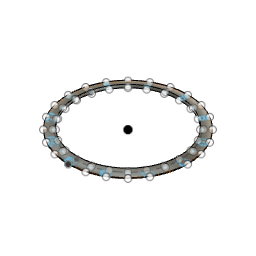
Bezel_Insert v4 (Autodesk Fusion 360 design; units mm, degrees)
Autodesk Fusion 360 part; units mm, degrees
note: some values were not read from the file. Set by a fixed rule: which sketch regions a step uses.
sketch "Sketch1" plane through (0, 0, 0) normal (0, 1, 0) x (1, 0, 0)
  line L0 (0, 0) -> (18.0594, 0) construction
  line L1 (18.0594, 0) -> (15.4305, 0)
  line L2 (18.0594, 0) -> (18.0594, -0.2032)
  arc A0 (15.5217, -0.9118) -> (18.0594, -0.2032) centre (15.4613, 4.2031) ccw
  line L3 (15.4305, 0) -> (15.5217, 0)
  line L4 (15.5217, 0) -> (15.5217, -0.9118)
  dimension "d2" = 15.4305
  dimension "d3" = 0.2032
  dimension "d5" = 2.6289
  constraint coincident L0.start origin
  constraint horizontal L0
  constraint vertical L2
  constraint coincident L1 L3.end
  constraint coincident L0 L3.end
  constraint perpendicular L3 L4
  measures "d2" distance of L0.start L1.end
  measures "d3" distance of L0.end L2.end
  measures "d5" distance of L0.end L1.end
revolve "Revolve1" add sketch "Sketch1" angle 360 about axis through (0, 0, 1.75) along (0, 0, 1)
sketch "Sketch2" plane through (0, 0, 0) normal (0, 0, -1) x (1, 0, 0)
  circle A0 centre (0, 0) radius 15.5217 construction
  circle A1 centre (0, 0) radius 18.0594 construction
  line L0 (0, 18.0594) -> (0, 15.5217) construction
  line L1 (-4.6741, 17.444) -> (-4.0173, 14.9928) construction
  line L2 (-9.0297, 15.6399) -> (-7.7609, 13.4422) construction
  line L3 (-12.7699, 12.7699) -> (-10.9755, 10.9755) construction
  line L4 (-15.6399, 9.0297) -> (-13.4422, 7.7609) construction
  line L5 (-17.444, 4.6741) -> (-14.9928, 4.0173) construction
  line L6 (-18.0594, 0) -> (-15.5217, 0) construction
  line L7 (-17.444, -4.6741) -> (-14.9928, -4.0173) construction
  line L8 (-15.6399, -9.0297) -> (-13.4422, -7.7609) construction
  line L9 (-12.7699, -12.7699) -> (-10.9755, -10.9755) construction
  line L10 (-9.0297, -15.6399) -> (-7.7609, -13.4422) construction
  line L11 (-4.6741, -17.444) -> (-4.0173, -14.9928) construction
  line L12 (0, -18.0594) -> (0, -15.5217) construction
  line L13 (4.6741, -17.444) -> (4.0173, -14.9928) construction
  line L14 (9.0297, -15.6399) -> (7.7609, -13.4422) construction
  line L15 (12.7699, -12.7699) -> (10.9755, -10.9755) construction
  line L16 (15.6399, -9.0297) -> (13.4422, -7.7609) construction
  line L17 (17.444, -4.6741) -> (14.9928, -4.0173) construction
  line L18 (18.0594, 0) -> (15.5217, 0) construction
  line L19 (17.444, 4.6741) -> (14.9928, 4.0173) construction
  line L20 (15.6399, 9.0297) -> (13.4422, 7.7609) construction
  line L21 (12.7699, 12.7699) -> (10.9755, 10.9755) construction
  line L22 (9.0297, 15.6399) -> (7.7609, 13.4422) construction
  line L23 (4.6741, 17.444) -> (4.0173, 14.9928) construction
  line L24 (-15.2263, 8.2238) -> (-15.3043, 8.2626)
  line L25 (-15.3043, 8.2626) -> (-15.499, 8.2622)
  line L26 (-15.499, 8.2622) -> (-15.6158, 8.2231)
  line L27 (-15.6158, 8.2231) -> (-15.7714, 8.1059)
  line L28 (-15.7714, 8.1059) -> (-15.9265, 7.794)
  line L29 (-15.9265, 7.794) -> (-15.9261, 7.5993)
  line L30 (-15.9261, 7.5993) -> (-15.887, 7.4825)
  line L31 (-15.887, 7.4825) -> (-15.7698, 7.327)
  line L32 (-15.7698, 7.327) -> (-15.6139, 7.2494)
  line L33 (-15.6139, 7.2494) -> (-15.4191, 7.2498)
  line L34 (-15.4191, 7.2498) -> (-15.1077, 7.2894)
  line L35 (-15.1077, 7.2894) -> (-13.94, 7.6811)
  line L36 (-13.94, 7.6811) -> (-14.4831, 6.5896)
  line L37 (-14.1837, 9.8328) -> (-14.2562, 9.8809)
  line L38 (-14.2562, 9.8809) -> (-14.4495, 9.9048)
  line L39 (-14.4495, 9.9048) -> (-14.5702, 9.8804)
  line L40 (-14.5702, 9.8804) -> (-14.7391, 9.7835)
  line L41 (-14.7391, 9.7835) -> (-14.9319, 9.4934)
  line L42 (-14.9319, 9.4934) -> (-14.9557, 9.3001)
  line L43 (-14.9557, 9.3001) -> (-14.9314, 9.1794)
  line L44 (-14.9314, 9.1794) -> (-14.8345, 9.0105)
  line L45 (-14.8345, 9.0105) -> (-14.6894, 8.9141)
  line L46 (-14.6894, 8.9141) -> (-14.4962, 8.8903)
  line L47 (-14.4962, 8.8903) -> (-14.1822, 8.8908)
  line L48 (-14.1822, 8.8908) -> (-12.9749, 9.1343)
  line L49 (-9.6456, 14.8241) -> (-9.3826, 14.9058)
  line L50 (-9.3826, 14.9058) -> (-9.0888, 14.7952)
  line L51 (-9.0888, 14.7952) -> (-8.764, 14.4924)
  line L52 (-8.764, 14.4924) -> (-8.6116, 14.2802)
  line L53 (-8.6116, 14.2802) -> (-8.4282, 13.8757)
  line L54 (-8.4282, 13.8757) -> (-8.4173, 13.5619)
  line L55 (-8.4173, 13.5619) -> (-8.5787, 13.3388)
  line L56 (-8.5787, 13.3388) -> (-8.7201, 13.2372)
  line L57 (-8.7201, 13.2372) -> (-8.9831, 13.1555)
  line L58 (-8.9831, 13.1555) -> (-9.277, 13.266)
  line L59 (-9.277, 13.266) -> (-9.6018, 13.5689)
  line L60 (-9.6018, 13.5689) -> (-9.7542, 13.7811)
  line L61 (-9.7542, 13.7811) -> (-9.9375, 14.1855)
  line L62 (-9.9375, 14.1855) -> (-9.9485, 14.4993)
  line L63 (-9.9485, 14.4993) -> (-9.7871, 14.7225)
  line L64 (-9.7871, 14.7225) -> (-9.6456, 14.8241)
  line L65 (-7.3643, 15.6598) -> (-7.406, 15.7363)
  line L66 (-7.406, 15.7363) -> (-7.5657, 15.8477)
  line L67 (-7.5657, 15.8477) -> (-7.6838, 15.8825)
  line L68 (-7.6838, 15.8825) -> (-7.8784, 15.8758)
  line L69 (-7.8784, 15.8758) -> (-8.1844, 15.7093)
  line L70 (-8.1844, 15.7093) -> (-8.2958, 15.5496)
  line L71 (-8.2958, 15.5496) -> (-8.3307, 15.4315)
  line L72 (-8.3307, 15.4315) -> (-8.3239, 15.2369)
  line L73 (-8.3239, 15.2369) -> (-8.2407, 15.0839)
  line L74 (-8.2407, 15.0839) -> (-8.081, 14.9725)
  line L75 (-8.081, 14.9725) -> (-7.8031, 14.8262)
  line L76 (-7.8031, 14.8262) -> (-6.622, 14.4774)
  line L77 (-6.622, 14.4774) -> (-7.693, 13.8948)
  line L78 (-0.8834, 17.6919) -> (-0.6167, 17.6234)
  line L79 (-0.6167, 17.6234) -> (-0.5176, 17.4558)
  line L80 (-0.5176, 17.4558) -> (-0.5053, 17.2821)
  line L81 (-0.5053, 17.2821) -> (-0.5799, 17.1022)
  line L82 (-0.5799, 17.1022) -> (-0.7475, 17.0031)
  line L83 (-0.7475, 17.0031) -> (-1.0889, 16.8917)
  line L84 (-1.0889, 16.8917) -> (-1.3434, 16.7864)
  line L85 (-1.3434, 16.7864) -> (-1.5049, 16.6004)
  line L86 (-1.5049, 16.6004) -> (-1.5795, 16.4206)
  line L87 (-1.5795, 16.4206) -> (-1.5611, 16.16)
  line L88 (-1.5611, 16.16) -> (-1.462, 15.9924)
  line L89 (-1.462, 15.9924) -> (-1.369, 15.9116)
  line L90 (-1.369, 15.9116) -> (-1.1022, 15.8431)
  line L91 (-1.1022, 15.8431) -> (-0.7547, 15.8677)
  line L92 (-0.7547, 15.8677) -> (-0.5003, 15.9729)
  line L93 (-0.5003, 15.9729) -> (-0.4195, 16.0659)
  line L94 (-0.4195, 16.0659) -> (-0.3449, 16.2458)
  line L95 (-0.3449, 16.2458) -> (-0.3633, 16.5064)
  line L96 (-0.3633, 16.5064) -> (-0.4624, 16.674)
  line L97 (-0.4624, 16.674) -> (-0.6484, 16.8355)
  line L98 (-0.6484, 16.8355) -> (-0.9152, 16.904)
  line L99 (-0.9152, 16.904) -> (-1.2688, 16.9663)
  line L100 (-1.2688, 16.9663) -> (-1.4486, 17.0409)
  line L101 (-1.4486, 17.0409) -> (-1.5478, 17.2085)
  line L102 (-1.5478, 17.2085) -> (-1.56, 17.3823)
  line L103 (-1.56, 17.3823) -> (-1.4854, 17.5621)
  line L104 (-1.4854, 17.5621) -> (-1.2309, 17.6674)
  line L105 (-1.2309, 17.6674) -> (-0.8834, 17.6919)
  line L106 (0.9655, 17.4038) -> (0.7154, 17.6757)
  line L107 (0.7154, 17.6757) -> (0.639, 15.8485)
  line L108 (7.357, 15.7798) -> (7.5057, 15.9056)
  line L109 (7.5057, 15.9056) -> (7.7801, 15.8828)
  line L110 (7.7801, 15.8828) -> (7.9402, 15.8142)
  line L111 (7.9402, 15.8142) -> (8.1461, 15.6313)
  line L112 (8.1461, 15.6313) -> (8.2033, 15.3225)
  line L113 (8.2033, 15.3225) -> (8.1118, 14.888)
  line L114 (8.1118, 14.888) -> (7.9404, 14.4877)
  line L115 (7.9404, 14.4877) -> (7.7231, 14.2018)
  line L116 (7.7231, 14.2018) -> (7.4944, 14.1103)
  line L117 (7.4944, 14.1103) -> (7.22, 14.1332)
  line L118 (7.22, 14.1332) -> (7.1399, 14.1675)
  line L119 (7.1399, 14.1675) -> (6.9341, 14.3504)
  line L120 (6.9341, 14.3504) -> (6.8426, 14.5791)
  line L121 (6.8426, 14.5791) -> (6.8654, 14.8535)
  line L122 (6.8654, 14.8535) -> (6.8997, 14.9336)
  line L123 (6.8997, 14.9336) -> (7.0827, 15.1394)
  line L124 (7.0827, 15.1394) -> (7.3113, 15.2309)
  line L125 (7.3113, 15.2309) -> (7.5858, 15.2081)
  line L126 (7.5858, 15.2081) -> (7.6658, 15.1738)
  line L127 (7.6658, 15.1738) -> (7.8717, 14.9909)
  line L128 (7.8717, 14.9909) -> (7.9632, 14.7622)
  line L129 (7.9632, 14.7622) -> (7.9404, 14.4877)
  line L130 (9.5325, 14.6777) -> (9.4346, 15.034)
  line L131 (9.4346, 15.034) -> (8.5306, 13.4442)
  line L132 (14.7542, 9.7576) -> (14.2009, 8.3652)
  line L133 (14.2009, 8.3652) -> (13.4935, 9.4633)
  line L134 (14.7542, 9.7576) -> (13.2168, 8.7672)
  line L135 (15.6269, 7.632) -> (15.745, 7.9821)
  line L136 (15.745, 7.9821) -> (14.1064, 7.1701)
  line L137 (17.3368, 0.2982) -> (17.4239, 0.3002)
  line L138 (17.4239, 0.3002) -> (17.5959, 0.3914)
  line L139 (17.5959, 0.3914) -> (17.6809, 0.4805)
  line L140 (17.6809, 0.4805) -> (17.7639, 0.6567)
  line L141 (17.7639, 0.6567) -> (17.7557, 1.005)
  line L142 (17.7557, 1.005) -> (17.6645, 1.177)
  line L143 (17.6645, 1.177) -> (17.5754, 1.262)
  line L144 (17.5754, 1.262) -> (17.3992, 1.345)
  line L145 (17.3992, 1.345) -> (17.2251, 1.3409)
  line L146 (17.2251, 1.3409) -> (17.053, 1.2497)
  line L147 (17.053, 1.2497) -> (16.7959, 1.0694)
  line L148 (16.7959, 1.0694) -> (15.9459, 0.1782)
  line L149 (15.9459, 0.1782) -> (15.9171, 1.3971)
  line L150 (17.3895, -1.1768) -> (17.6728, -0.9396)
  line L151 (17.6728, -0.9396) -> (15.8512, -0.7778)
  line L152 (15.7537, -8.1665) -> (15.5641, -8.3662)
  line L153 (15.5641, -8.3662) -> (15.2536, -8.4132)
  line L154 (15.2536, -8.4132) -> (14.8223, -8.3074)
  line L155 (14.8223, -8.3074) -> (14.5857, -8.1967)
  line L156 (14.5857, -8.1967) -> (14.2283, -7.9332)
  line L157 (14.2283, -7.9332) -> (14.0655, -7.6647)
  line L158 (14.0655, -7.6647) -> (14.0974, -7.3911)
  line L159 (14.0974, -7.3911) -> (14.1713, -7.2334)
  line L160 (14.1713, -7.2334) -> (14.3609, -7.0337)
  line L161 (14.3609, -7.0337) -> (14.6714, -6.9867)
  line L162 (14.6714, -6.9867) -> (15.1027, -7.0925)
  line L163 (15.1027, -7.0925) -> (15.3393, -7.2032)
  line L164 (15.3393, -7.2032) -> (15.6967, -7.4667)
  line L165 (15.6967, -7.4667) -> (15.8595, -7.7352)
  line L166 (15.8595, -7.7352) -> (15.8276, -8.0088)
  line L167 (15.8276, -8.0088) -> (15.7537, -8.1665)
  line L168 (14.5652, -9.7204) -> (14.9245, -9.6342)
  line L169 (14.9245, -9.6342) -> (13.3655, -8.6782)
  line L170 (8.7046, -15.4101) -> (8.4366, -15.4732)
  line L171 (8.4366, -15.4732) -> (8.271, -15.3707)
  line L172 (8.271, -15.3707) -> (8.1795, -15.2225)
  line L173 (8.1795, -15.2225) -> (8.1621, -15.0286)
  line L174 (8.1621, -15.0286) -> (8.2646, -14.863)
  line L175 (8.2646, -14.863) -> (8.5153, -14.6059)
  line L176 (8.5153, -14.6059) -> (8.6918, -14.3946)
  line L177 (8.6918, -14.3946) -> (8.7486, -14.1549)
  line L178 (8.7486, -14.1549) -> (8.7312, -13.9609)
  line L179 (8.7312, -13.9609) -> (8.594, -13.7386)
  line L180 (8.594, -13.7386) -> (8.4284, -13.6361)
  line L181 (8.4284, -13.6361) -> (8.3085, -13.6078)
  line L182 (8.3085, -13.6078) -> (8.0405, -13.6709)
  line L183 (8.0405, -13.6709) -> (7.744, -13.8539)
  line L184 (7.744, -13.8539) -> (7.5675, -14.0652)
  line L185 (7.5675, -14.0652) -> (7.5391, -14.185)
  line L186 (7.5391, -14.185) -> (7.5565, -14.379)
  line L187 (7.5565, -14.379) -> (7.6937, -14.6013)
  line L188 (7.6937, -14.6013) -> (7.8593, -14.7038)
  line L189 (7.8593, -14.7038) -> (8.099, -14.7605)
  line L190 (8.099, -14.7605) -> (8.3671, -14.6974)
  line L191 (8.3671, -14.6974) -> (8.7092, -14.5885)
  line L192 (8.7092, -14.5885) -> (8.9032, -14.5711)
  line L193 (8.9032, -14.5711) -> (9.0688, -14.6736)
  line L194 (9.0688, -14.6736) -> (9.1603, -14.8218)
  line L195 (9.1603, -14.8218) -> (9.1776, -15.0158)
  line L196 (9.1776, -15.0158) -> (9.0011, -15.2271)
  line L197 (9.0011, -15.2271) -> (8.7046, -15.4101)
  line L198 (0.5376, -17.3918) -> (0.4634, -17.5718)
  line L199 (0.4634, -17.5718) -> (0.2092, -17.6777)
  line L200 (0.2092, -17.6777) -> (0.0355, -17.6904)
  line L201 (0.0355, -17.6904) -> (-0.2314, -17.6225)
  line L202 (-0.2314, -17.6225) -> (-0.4241, -17.3746)
  line L203 (-0.4241, -17.3746) -> (-0.5427, -16.9467)
  line L204 (-0.5427, -16.9467) -> (-0.5744, -16.5124)
  line L205 (-0.5744, -16.5124) -> (-0.5129, -16.1587)
  line L206 (-0.5129, -16.1587) -> (-0.3518, -15.9723)
  line L207 (-0.3518, -15.9723) -> (-0.0976, -15.8664)
  line L208 (-0.0976, -15.8664) -> (-0.0108, -15.8601)
  line L209 (-0.0108, -15.8601) -> (0.2561, -15.9279)
  line L210 (0.2561, -15.9279) -> (0.4425, -16.0889)
  line L211 (0.4425, -16.0889) -> (0.5484, -16.3432)
  line L212 (0.5484, -16.3432) -> (0.5547, -16.43)
  line L213 (0.5547, -16.43) -> (0.4869, -16.6969)
  line L214 (0.4869, -16.6969) -> (0.3259, -16.8833)
  line L215 (0.3259, -16.8833) -> (0.0717, -16.9892)
  line L216 (0.0717, -16.9892) -> (-0.0152, -16.9955)
  line L217 (-0.0152, -16.9955) -> (-0.2821, -16.9277)
  line L218 (-0.2821, -16.9277) -> (-0.4685, -16.7667)
  line L219 (-0.4685, -16.7667) -> (-0.5744, -16.5124)
  line L220 (-8.7289, -15.4091) -> (-8.9167, -13.9226)
  line L221 (-8.9167, -13.9226) -> (-7.767, -14.5426)
  line L222 (-8.7289, -15.4091) -> (-7.8609, -13.7994)
  line L223 (-15.2459, -8.1332) -> (-15.322, -8.1756)
  line L224 (-15.322, -8.1756) -> (-15.4316, -8.3365)
  line L225 (-15.4316, -8.3365) -> (-15.4653, -8.455)
  line L226 (-15.4653, -8.455) -> (-15.4565, -8.6495)
  line L227 (-15.4565, -8.6495) -> (-15.2868, -8.9538)
  line L228 (-15.2868, -8.9538) -> (-15.1259, -9.0634)
  line L229 (-15.1259, -9.0634) -> (-15.0074, -9.0971)
  line L230 (-15.0074, -9.0971) -> (-14.8129, -9.0883)
  line L231 (-14.8129, -9.0883) -> (-14.6608, -9.0034)
  line L232 (-14.6608, -9.0034) -> (-14.5511, -8.8425)
  line L233 (-14.5511, -8.8425) -> (-14.4078, -8.5631)
  line L234 (-14.4078, -8.5631) -> (-14.0715, -7.3784)
  line L235 (-14.0715, -7.3784) -> (-13.4775, -8.4431)
  line L236 (-12.9749, 9.1343) -> (-13.6246, 8.0624)
  circle A2 centre (0, 0) radius 15.748 construction
  line L237 (17.444, 4.6741) -> (17.2214, 4.6145) construction
  circle A3 centre (0, 0) radius 17.8289 construction
  line L238 (-17.682, -0.7501) -> (-15.9065, 0)
  line L239 (-17.682, 0.7501) -> (-15.9065, 0)
  line L240 (-17.682, -0.7501) -> (-17.682, 0.7501)
  circle A4 centre (-15.5839, -4.1757) radius 0.174
  circle A5 centre (-11.4082, -11.4082) radius 0.174
  circle A6 centre (-4.1757, -15.5839) radius 0.174
  circle A7 centre (4.1757, -15.5839) radius 0.174
  circle A8 centre (11.4082, -11.4082) radius 0.174
  circle A9 centre (15.5839, -4.1757) radius 0.174
  circle A10 centre (15.5839, 4.1757) radius 0.174
  circle A11 centre (11.4082, 11.4082) radius 0.174
  circle A12 centre (4.1757, 15.5839) radius 0.174
  circle A13 centre (-4.1757, 15.5839) radius 0.174
  circle A14 centre (-11.4082, 11.4082) radius 0.174
  circle A15 centre (-15.5839, 4.1757) radius 0.174
  dimension "d7" = 360
  dimension "d11" = 31.496
  dimension "d13" = 360
  constraint coincident A1 L0.start
  constraint coincident A0 L0.end
  constraint coincident A0.centre A1.centre
  constraint coincident L19 L237.end
  constraint concentric A2 A3
  constraint coincident L237.end A3
  constraint coincident L6 L238.end
  constraint symmetric L6 L238.start L239.start
  constraint symmetric L6 L238.end L239.end
  constraint coincident L7 A4.centre
  measures "d11" diameter of A2
equation "d2 = ( 1.215 / 2 ) * 1 in"
